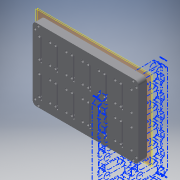
# Autodesk Inventor part: 02_Omniscope_lid_bottom
Saved by Autodesk Inventor 2019.4 (Build 234330000, 330)
## iProperties
Created: 2021-09-27
Part Number: 02_Omniscope_lid_bottom
Material: Generic
Document SubType Name: Modeling
Designer: diederichbenedict
Density: 1 g/cm^3
Appearance: Default
Author: diederichbenedict
Autodesk Inventor part; units mm, degrees
ref_plane "YZ Plane" through (0, 0, 0) normal (1, 0, 0) x (0, 1, 0)
ref_plane "XZ Plane" through (0, 0, 0) normal (0, 1, 0) x (-1, 0, 0)
ref_plane "XY Plane" through (0, 0, 0) normal (0, 0, 1) x (1, 0, 0)
ref_plane "Work Plane1" through (0, 0, 0) normal (0, 0, 1) x (1, 0, 0)
ref_plane "Work Plane2" through (0, 0, 1.8307) normal (0, 0, 1) x (1, 0, 0)
sketch "Sketch2" plane through (0, 0, 1.8307) normal (0, 0, 1) x (1, 0, 0)
  line L0 (-53.8717, 35.9824) -> (54.9283, 35.9824) projected
  line L1 (54.9283, 35.9824) -> (54.9283, -35.8176) projected
  line L2 (54.9283, -35.8176) -> (-53.8717, -35.8176) projected
  line L3 (-53.8717, -35.8176) -> (-53.8717, 35.9824) projected
  arc A0 (55.0283, -39.9176) -> (59.0283, -35.9176) centre (55.0283, -35.9176) ccw projected
  line L4 (59.0283, 36.0824) -> (59.0283, -35.9176) projected
  arc A1 (59.0283, 36.0824) -> (55.0283, 40.0824) centre (55.0283, 36.0824) ccw projected
  line L5 (-53.9717, 40.0824) -> (55.0283, 40.0824) projected
  arc A2 (-53.9717, 40.0824) -> (-57.9717, 36.0824) centre (-53.9717, 36.0824) ccw projected
  line L6 (-57.9717, -35.9176) -> (-57.9717, 36.0824) projected
  arc A3 (-57.9717, -35.9176) -> (-53.9717, -39.9176) centre (-53.9717, -35.9176) ccw projected
  line L7 (55.0283, -39.9176) -> (-53.9717, -39.9176) projected
  circle A4 centre (-51.9717, 38.0824) radius 1.35 projected
  circle A5 centre (56.5283, 33.5824) radius 1.35 projected
  circle A6 centre (53.0283, -37.9176) radius 1.35 projected
  circle A7 centre (-55.4717, -33.4176) radius 1.35 projected
  circle A8 centre (-51.9717, -37.9176) radius 1.35 projected
  circle A9 centre (56.5283, -33.4176) radius 1.35 projected
  circle A10 centre (53.0283, 38.0824) radius 1.35 projected
  circle A11 centre (-55.4717, 33.5824) radius 1.35 projected
  point P0 (0, 0)
extrude "Extrusion1" add sketch "Sketch2" along normal blind 9.3 contours L0 L1 L2 L3 | L7 A3 L6 A2 L5 A1 L4 A0
sketch "Sketch3" plane through (0, 0, 11.1307) normal (0, 0, 1) x (1, 0, 0)
  circle A0 centre (-55.4717, 33.5824) radius 1.35 projected
  circle A1 centre (53.0283, 38.0824) radius 1.35 projected
  circle A2 centre (56.5283, -33.4176) radius 1.35 projected
  circle A3 centre (-51.9717, -37.9176) radius 1.35 projected
  circle A4 centre (-55.4717, -33.4176) radius 1.35 projected
  circle A5 centre (53.0283, -37.9176) radius 1.35 projected
  circle A6 centre (56.5283, 33.5824) radius 1.35 projected
  circle A7 centre (-51.9717, 38.0824) radius 1.35 projected
  arc A8 (55.0283, -39.9176) -> (59.0283, -35.9176) centre (55.0283, -35.9176) ccw projected
  line L0 (59.0283, -35.9176) -> (59.0283, 36.0824) projected
  arc A9 (59.0283, 36.0824) -> (55.0283, 40.0824) centre (55.0283, 36.0824) ccw projected
  line L1 (55.0283, 40.0824) -> (-53.9717, 40.0824) projected
  arc A10 (-53.9717, 40.0824) -> (-57.9717, 36.0824) centre (-53.9717, 36.0824) ccw projected
  line L2 (-57.9717, 36.0824) -> (-57.9717, -35.9176) projected
  arc A11 (-57.9717, -35.9176) -> (-53.9717, -39.9176) centre (-53.9717, -35.9176) ccw projected
  line L3 (-53.9717, -39.9176) -> (55.0283, -39.9176) projected
  line L4 (-49.5298, 12.2324) -> (-47.8298, 12.2324) projected
  line L5 (-47.8298, 12.2324) -> (-47.8298, 23.7324) projected
  line L6 (-47.8298, 23.7324) -> (-49.5298, 23.7324) projected
  line L7 (-49.5298, 23.7324) -> (-49.5298, 12.2324) projected
  circle A12 centre (-39.0634, 1.6824) radius 1 projected
  circle A13 centre (-39.0634, 34.2824) radius 1 projected
  circle A14 centre (-50.8634, 34.2824) radius 1 projected
  circle A15 centre (-50.8634, 1.6824) radius 1 projected
  line L8 (-53.8634, 34.8824) -> (-53.8634, 1.0824) projected
  line L9 (-52.8634, 35.8824) -> (-53.8634, 34.8824) projected
  line L10 (-37.0634, 35.8824) -> (-52.8634, 35.8824) projected
  line L11 (-36.0634, 34.8824) -> (-37.0634, 35.8824) projected
  line L12 (-36.0634, 1.0824) -> (-36.0634, 34.8824) projected
  line L13 (-37.0634, 0.0824) -> (-36.0634, 1.0824) projected
  line L14 (-52.8634, 0.0824) -> (-37.0634, 0.0824) projected
  line L15 (-53.8634, 1.0824) -> (-52.8634, 0.0824) projected
  circle A16 centre (-50.9634, 6.9824) radius 1.2902 construction
  circle A17 centre (-38.9634, 6.9824) radius 1.5 construction
  circle A18 centre (-50.9634, 28.9824) radius 1.2902 construction
  circle A19 centre (-38.9634, 28.9824) radius 1.2902 construction
  circle A20 centre (-38.9634, 28.9824) radius 1.45
  circle A21 centre (-38.9634, 6.9824) radius 1.45
  line L16 (-49.5298, 12.2324) -> (-47.8298, 12.2324) projected
  line L17 (-47.8298, 12.2324) -> (-47.8298, 23.7324) projected
  line L18 (-47.8298, 23.7324) -> (-49.5298, 23.7324) projected
  line L19 (-49.5298, 23.7324) -> (-49.5298, 12.2324) projected
  circle A22 centre (-39.0634, 1.6824) radius 1 projected
  circle A23 centre (-39.0634, 34.2824) radius 1 projected
  circle A24 centre (-50.8634, 34.2824) radius 1 projected
  circle A25 centre (-50.8634, 1.6824) radius 1 projected
  line L20 (-53.8634, 34.8824) -> (-53.8634, 1.0824) projected
  line L21 (-52.8634, 35.8824) -> (-53.8634, 34.8824) projected
  line L22 (-37.0634, 35.8824) -> (-52.8634, 35.8824) projected
  line L23 (-36.0634, 34.8824) -> (-37.0634, 35.8824) projected
  line L24 (-36.0634, 1.0824) -> (-36.0634, 34.8824) projected
  line L25 (-37.0634, 0.0824) -> (-36.0634, 1.0824) projected
  line L26 (-52.8634, 0.0824) -> (-37.0634, 0.0824) projected
  line L27 (-53.8634, 1.0824) -> (-52.8634, 0.0824) projected
  circle A26 centre (-48.6798, 5.2824) radius 0.375 projected
  circle A27 centre (-48.6798, 7.8224) radius 0.375 projected
  circle A28 centre (-48.6798, 10.3624) radius 0.375 projected
  circle A29 centre (-48.6798, 12.9024) radius 0.375 projected
  circle A30 centre (-48.6798, 15.4424) radius 0.375 projected
  circle A31 centre (-48.6798, 17.9824) radius 0.375 projected
  circle A32 centre (-48.6798, 20.5224) radius 0.375 projected
  circle A33 centre (-48.6798, 23.0624) radius 0.375 projected
  circle A34 centre (-48.6798, 25.6024) radius 0.375 projected
  circle A35 centre (-48.6798, 28.1424) radius 0.375 projected
  line L28 (-49.8648, 3.7524) -> (-47.4948, 3.7524) projected
  line L29 (-47.4948, 3.7524) -> (-47.4948, 29.5924) projected
  line L30 (-47.4948, 29.5924) -> (-49.8648, 29.5924) projected
  line L31 (-49.8648, 29.5924) -> (-49.8648, 3.7524) projected
  line L32 (-47.2948, 29.7924) -> (-47.2948, 3.5524)
  line L33 (-47.2948, 3.5524) -> (-50.0648, 3.5524)
  line L34 (-50.0648, 3.5524) -> (-50.0648, 29.7924)
  line L35 (-50.0648, 29.7924) -> (-47.2948, 29.7924)
  line L36 (-47.6948, 29.3924) -> (-47.6948, 3.9524)
  line L37 (-47.6948, 3.9524) -> (-49.6648, 3.9524)
  line L38 (-49.6648, 3.9524) -> (-49.6648, 29.3924)
  line L39 (-49.6648, 29.3924) -> (-47.6948, 29.3924)
  circle A36 centre (-50.9634, 28.9824) radius 1.45
  circle A37 centre (-50.8634, 1.6824) radius 1.45
  circle A38 centre (-50.9634, 6.9824) radius 1.45
  point P0 (0, 0)
  dimension "d7" = 2.9
  dimension "d8" = 2.9
  dimension "d35" = 0.2
  dimension "d36" = 0.2
  dimension "d39" = 2.9
  dimension "d40" = 2.9
  dimension "d41" = 2.9
  constraints: 16 end point, 5 centre point, 3 coincident, 6 other
  measures "d7" diameter of A20
  measures "d8" diameter of A21
  measures "d35" distance between parallel lines of L29 L32
  measures "d36" distance between parallel lines of L29 L36
  measures "d39" diameter of A36
  measures "d40" diameter of A37
  measures "d41" diameter of A38
extrude "Extrusion2" cut sketch "Sketch3" against normal through all contours L7 L6 L5 L4 | A20 | A21 | A26 | A27 | A28 | A29 | A30 | A31 | A32 | A33 | A34 | A35 | A38 L34 L31 | L31 A38 L38 | A38 L34 | A38 L38 A36 L39 L36 L37 | L38 A38 | A36 L39 L38 L31 L30 | L30 L31 A36 L34 L35 | A36 L38 L39 | L35 L34 A36
sketch "Sketch4" plane through (0, 0, 11.1307) normal (0, 0, 1) x (1, 0, 0)
  circle A0 centre (-38.9634, 6.9824) radius 1.45 projected
  circle A1 centre (-38.9634, 28.9824) radius 1.45 projected
  line L0 (-49.5726, 29.3924) -> (-47.6948, 29.3924) projected
  line L1 (-47.6948, 29.3924) -> (-47.6948, 3.9524) projected
  line L2 (-47.6948, 3.9524) -> (-49.6648, 3.9524) projected
  line L3 (-49.6648, 3.9524) -> (-49.6648, 6.3375) projected
  circle A2 centre (-55.4717, 33.5824) radius 1.35 projected
  circle A3 centre (53.0283, 38.0824) radius 1.35 projected
  circle A4 centre (56.5283, -33.4176) radius 1.35 projected
  circle A5 centre (-51.9717, -37.9176) radius 1.35 projected
  circle A6 centre (-55.4717, -33.4176) radius 1.35 projected
  circle A7 centre (53.0283, -37.9176) radius 1.35 projected
  circle A8 centre (56.5283, 33.5824) radius 1.35 projected
  circle A9 centre (-51.9717, 38.0824) radius 1.35 projected
  arc A10 (55.0283, -39.9176) -> (59.0283, -35.9176) centre (55.0283, -35.9176) ccw projected
  line L4 (59.0283, -35.9176) -> (59.0283, 36.0824) projected
  arc A11 (59.0283, 36.0824) -> (55.0283, 40.0824) centre (55.0283, 36.0824) ccw projected
  line L5 (55.0283, 40.0824) -> (-53.9717, 40.0824) projected
  arc A12 (-53.9717, 40.0824) -> (-57.9717, 36.0824) centre (-53.9717, 36.0824) ccw projected
  line L6 (-57.9717, 36.0824) -> (-57.9717, -35.9176) projected
  arc A13 (-57.9717, -35.9176) -> (-53.9717, -39.9176) centre (-53.9717, -35.9176) ccw projected
  line L7 (-53.9717, -39.9176) -> (55.0283, -39.9176) projected
  line L8 (-47.8948, 4.1524) -> (-47.8948, 29.1924)
  line L9 (-47.8948, 29.1924) -> (-49.4648, 29.1924)
  line L10 (-49.4648, 29.1924) -> (-49.4648, 4.1524)
  line L11 (-49.4648, 4.1524) -> (-47.8948, 4.1524)
  arc A14 (-49.6648, 7.6273) -> (-49.6648, 6.3375) centre (-50.9634, 6.9824) ccw projected
  line L12 (-49.6648, 7.6273) -> (-49.6648, 28.3375) projected
  arc A15 (-49.5726, 29.3924) -> (-49.6648, 28.3375) centre (-50.9634, 28.9824) ccw projected
  line L13 (-47.6948, 29.3924) -> (-49.6648, 29.3924)
  line L14 (-49.6648, 29.3924) -> (-49.6648, 3.9524)
  line L15 (-49.6648, 3.9524) -> (-47.6948, 3.9524)
  line L16 (-47.6948, 3.9524) -> (-47.6948, 29.3924)
  point P0 (0, 0)
  dimension "d37" = 0.2
  constraints: 16 end point, 2 parallel, 1 horizontal, 1 perpendicular, 3 other
  measures "d37" distance between parallel lines of L1 L8
extrude "Extrusion3" add sketch "Sketch4" against normal blind 1 contours L0 L1 L2 L3 L14 L12 L13
pattern_linear "Rectangular Pattern2" count 6 spacing 18 along (1, 0, 0) count 2 spacing 36 along (0, -1, 0) of "Extrusion2", "Extrusion3"
shell "Shell2" [suppressed]
body "Solid1"
